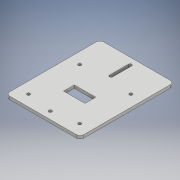
# Autodesk Inventor part: Адаптер для считывателя Bolid Proxy-2MA часть 2
Saved by Autodesk Inventor 2018 (Build 220112000, 112)
## iProperties
Created: 2019-06-30
Part Number: Адаптер для считывателя Bolid Proxy-2MA часть 2
Material: Типовые
Document SubType Name: Modeling
Designer: KV33_HP1
Density: 1 g/cm^3
Appearance: По умолчанию
Author: KV33_HP1
Autodesk Inventor part; units mm, degrees
ref_plane "YZ Plane" through (0, 0, 0) normal (1, 0, 0) x (0, 1, 0)
ref_plane "XZ Plane" through (0, 0, 0) normal (0, 1, 0) x (-1, 0, 0)
ref_plane "XY Plane" through (0, 0, 0) normal (0, 0, 1) x (1, 0, 0)
sketch "Эскиз1" plane through (0, 0, 0) normal (0, 0, 1) x (1, 0, 0)
  line L0 (5, 0) -> (92, 0)
  line L1 (97, 5) -> (97, 118)
  line L2 (92, 123) -> (5, 123)
  line L3 (0, 118) -> (0, 5)
  arc A0 (5, 123) -> (0, 118) centre (5, 118) ccw
  arc A1 (97, 118) -> (92, 123) centre (92, 118) ccw
  arc A2 (92, 0) -> (97, 5) centre (92, 5) ccw
  arc A3 (0, 5) -> (5, 0) centre (5, 5) ccw
  arc A4 (46.5, 89) -> (50.5, 89) centre (48.5, 89) ccw
  arc A5 (50.5, 114) -> (46.5, 114) centre (48.5, 114) ccw
  line L4 (46.5, 89) -> (46.5, 114)
  line L5 (50.5, 114) -> (50.5, 89)
  circle A6 centre (48.5, 9.5) radius 2
  line L6 (34.5, 41) -> (62.5, 41)
  line L7 (62.5, 41) -> (62.5, 55)
  line L8 (62.5, 55) -> (34.5, 55)
  line L9 (34.5, 55) -> (34.5, 41)
  circle A7 centre (15, 14.5) radius 2
  circle A8 centre (15, 81.5) radius 2
  circle A9 centre (82, 81.5) radius 2
  circle A10 centre (82, 14.5) radius 2
  point P0 (0, 0)
  point P1 (97, 123)
  point P2 (0, 123)
  dimension "d10" = 5
  dimension "d21" = 4
  dimension "d22" = 4
  dimension "d23" = 4
  dimension "d29" = 28
  dimension "d30" = 14
  constraints: 20 end point, 12 point on circle, 11 centre point, 10 tangent, 6 point on line, 5 parallel, 3 equal radius, 2 horizontal, 2 perpendicular, 1 coincident, 1 vertical
  measures "d10" radius of A0
  measures "d21" diameter of A4
  measures "d22" diameter of A5
  measures "d23" diameter of A6
  measures "d29" distance of L8.end L7.end
  measures "d30" distance of L7.end L6.end
extrude "Выдавливание2" add sketch "Эскиз1" along normal blind 4
